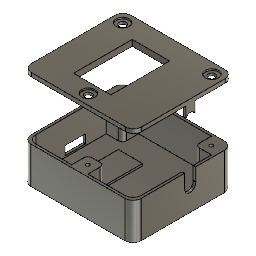
ScopeControl-fusion360 (Autodesk Fusion 360 design; units mm, degrees)
Autodesk Fusion 360 part; units mm, degrees
sketch "Sketch1" plane through (0, 0, 0) normal (0, 0, 1) x (1, 0, 0)
  line L0 (0, 0) -> (54.6, 0)
  line L1 (54.6, 0) -> (54.6, -49.3)
  line L2 (54.6, -49.3) -> (0, -49.3)
  line L3 (0, -49.3) -> (0, 0)
  dimension "d1" = 54.6
  dimension "d2" = 49.3
  constraint horizontal L0
  constraint vertical L1
  constraint horizontal L2
  constraint vertical L3
  constraint coincident L0.start L3.end
  measures "d1" distance of L0.start L0.end
  measures "d2" distance of L0.start L2.end
extrude "Extrude1" add sketch "Sketch1" along normal blind 1.25 makes body 1
sketch "Sketch2" plane through (0, 0, 1.25) normal (0, 0, 1) x (-1, 0, 0)
  line L0 (0, 49.3) -> (-54.6, 49.3)
  line L1 (-54.6, 49.3) -> (-54.6, 0)
  line L2 (-54.6, 0) -> (0, 0)
  line L3 (0, 0) -> (0, 49.3)
  line L4 (-1.25, 48.05) -> (-53.35, 48.05)
  line L5 (-53.35, 48.05) -> (-53.35, 1.25)
  line L6 (-53.35, 1.25) -> (-1.25, 1.25)
  line L7 (-1.25, 1.25) -> (-1.25, 48.05)
  dimension "d5" = -1.25
extrude "Extrude2" add sketch "Sketch2" along normal blind 17.5 bodies 1
sketch "Sketch3" plane through (0, 0, 1.25) normal (0, 0, 1) x (-1, 0, 0)
  line L0 (-1.25, 48.05) -> (-53.35, 48.05)
  line L1 (-53.35, 48.05) -> (-53.35, 1.25)
  line L2 (-53.35, 1.25) -> (-1.25, 1.25)
  line L3 (-1.25, 1.25) -> (-1.25, 48.05)
  line L4 (-1.25, 1.25) -> (-9.25, 1.25)
  line L5 (-9.25, 1.25) -> (-9.25, 9.25)
  line L6 (-9.25, 9.25) -> (-1.25, 9.25)
  line L7 (-1.25, 9.25) -> (-1.25, 1.25)
  dimension "d8" = 8
  dimension "d9" = 8
  constraint horizontal L4
  constraint vertical L5
  constraint horizontal L6
  constraint vertical L7
  constraint coincident L2.end L3.start
  measures "d8" distance of L2.end L4.end
  measures "d9" distance of L2.end L6.end
extrude "Extrude3" add sketch "Sketch3" along normal blind 17.5 contours L2 L3 L4 L5 L6 L7 bodies 1
sketch "Sketch4" plane through (0, 0, 1.25) normal (0, 0, 1) x (-1, 0, 0)
  line L0 (-9.25, 1.25) -> (-9.25, 9.25)
  line L1 (-9.25, 9.25) -> (-1.25, 9.25)
  line L2 (-1.25, 9.25) -> (-1.25, 48.05)
  line L3 (-1.25, 48.05) -> (-53.35, 48.05)
  line L4 (-53.35, 48.05) -> (-53.35, 1.25)
  line L5 (-53.35, 1.25) -> (-9.25, 1.25)
  line L6 (-53.35, 1.25) -> (-45.35, 1.25)
  line L7 (-45.35, 1.25) -> (-45.35, 9.25)
  line L8 (-45.35, 9.25) -> (-53.35, 9.25)
  line L9 (-53.35, 9.25) -> (-53.35, 1.25)
  dimension "d12" = 8
  dimension "d13" = 8
  constraint horizontal L6
  constraint vertical L7
  constraint horizontal L8
  constraint vertical L9
  constraint coincident L4.end L5.start
  measures "d12" distance of L4.end L6.end
  measures "d13" distance of L4.end L8.end
extrude "Extrude4" add sketch "Sketch4" along normal blind 17.5 contours L4 L5 L6 L7 L8 L9 bodies 1
sketch "Sketch5" plane through (0, 0, 1.25) normal (0, 0, 1) x (-1, 0, 0)
  line L0 (-45.35, 9.25) -> (-45.35, 1.25)
  line L1 (-45.35, 1.25) -> (-9.25, 1.25)
  line L2 (-9.25, 1.25) -> (-9.25, 9.25)
  line L3 (-9.25, 9.25) -> (-1.25, 9.25)
  line L4 (-1.25, 9.25) -> (-1.25, 48.05)
  line L5 (-1.25, 48.05) -> (-53.35, 48.05)
  line L6 (-53.35, 48.05) -> (-53.35, 9.25)
  line L7 (-53.35, 9.25) -> (-45.35, 9.25)
  line L8 (-22.9932, 48.05) -> (-30.9932, 48.05)
  line L9 (-30.9932, 48.05) -> (-30.9932, 40.05)
  line L10 (-30.9932, 40.05) -> (-22.9932, 40.05)
  line L11 (-22.9932, 40.05) -> (-22.9932, 48.05)
  dimension "d16" = 8
  dimension "d17" = 8
  constraint horizontal L8
  constraint vertical L9
  constraint horizontal L10
  constraint vertical L11
  constraint coincident L5 L8.start
  measures "d16" distance of L8.start L8.end
  measures "d17" distance of L8.start L10.end
extrude "Extrude5" add sketch "Sketch5" along normal blind 17.5 contours L5 L8 L9 L10 L11 bodies 1
sketch "Sketch6" plane through (0, 0, 0) normal (-1, 0, 0) x (0, -1, 0)
  line L0 (0, 0) -> (49.3, 0)
  line L1 (49.3, 0) -> (49.3, 18.75)
  line L2 (49.3, 18.75) -> (0, 18.75)
  line L3 (0, 18.75) -> (0, 0)
  line L4 (19.5046, 2.0157) -> (29.5046, 2.0157)
  line L5 (29.5046, 2.0157) -> (29.5046, 6.3157)
  line L6 (29.5046, 6.3157) -> (19.5046, 6.3157)
  line L7 (19.5046, 6.3157) -> (19.5046, 2.0157)
  dimension "d20" = 10
  dimension "d21" = 4.3
  constraint horizontal L4
  constraint vertical L5
  constraint horizontal L6
  constraint vertical L7
  measures "d20" distance of L4.start L4.end
  measures "d21" distance of L4.start L6.end
extrude "Extrude6" cut sketch "Sketch6" against normal blind 2 contours L4 L5 L6 L7 bodies 1
sketch "Sketch7" plane through (54.6, 0, 0) normal (1, 0, 0) x (0, 1, 0)
  line L0 (-49.3, 0) -> (0, 0)
  line L1 (0, 0) -> (0, 18.75)
  line L2 (0, 18.75) -> (-49.3, 18.75)
  line L3 (-49.3, 18.75) -> (-49.3, 0)
  circle A0 centre (-21.0556, 11.4278) radius 2.75
  dimension "d24" = 5.5
  measures "d24" diameter of A0
extrude "Extrude7" cut sketch "Sketch7" against normal blind 2 contours A0 bodies 1
sketch "Sketch8" plane through (0, 0, 1.25) normal (0, 0, 1) x (-1, 0, 0)
  line L0 (-30.9932, 40.05) -> (-30.9932, 48.05)
  line L1 (-30.9932, 48.05) -> (-53.35, 48.05)
  line L2 (-53.35, 48.05) -> (-53.35, 9.25)
  line L3 (-53.35, 9.25) -> (-45.35, 9.25)
  line L4 (-45.35, 9.25) -> (-45.35, 1.25)
  line L5 (-45.35, 1.25) -> (-9.25, 1.25)
  line L6 (-9.25, 1.25) -> (-9.25, 9.25)
  line L7 (-9.25, 9.25) -> (-1.25, 9.25)
  line L8 (-1.25, 9.25) -> (-1.25, 48.05)
  line L9 (-1.25, 48.05) -> (-22.9932, 48.05)
  line L10 (-22.9932, 48.05) -> (-22.9932, 40.05)
  line L11 (-22.9932, 40.05) -> (-30.9932, 40.05)
  line L12 (-12, 14) -> (-24, 14)
  line L13 (-24, 14) -> (-24, 36)
  line L14 (-24, 36) -> (-12, 36)
  line L15 (-12, 36) -> (-12, 14)
  dimension "d27" = 12
  dimension "d28" = 22
  constraint horizontal L12
  constraint vertical L13
  constraint horizontal L14
  constraint vertical L15
  measures "d27" distance of L12.start L12.end
  measures "d28" distance of L12.start L14.end
extrude "Extrude8" add sketch "Sketch8" along normal blind 1 contours L12 L13 L14 L15 bodies 1
sketch "Sketch9" plane through (0, 0, 18.75) normal (0, 0, 1) x (-1, 0, 0)
  line L0 (-1.25, 48.05) -> (-1.25, 9.25)
  line L1 (-1.25, 9.25) -> (-9.25, 9.25)
  line L2 (-9.25, 9.25) -> (-9.25, 1.25)
  line L3 (-9.25, 1.25) -> (-45.35, 1.25)
  line L4 (-45.35, 1.25) -> (-45.35, 9.25)
  line L5 (-45.35, 9.25) -> (-53.35, 9.25)
  line L6 (-53.35, 9.25) -> (-53.35, 48.05)
  line L7 (-53.35, 48.05) -> (-30.9932, 48.05)
  line L8 (-30.9932, 48.05) -> (-30.9932, 40.05)
  line L9 (-30.9932, 40.05) -> (-22.9932, 40.05)
  line L10 (-22.9932, 40.05) -> (-22.9932, 48.05)
  line L11 (-22.9932, 48.05) -> (-1.25, 48.05)
  line L12 (0, 0) -> (0, 49.3)
  line L13 (0, 49.3) -> (-54.6, 49.3)
  line L14 (-54.6, 49.3) -> (-54.6, 0)
  line L15 (-54.6, 0) -> (0, 0)
  line L16 (0, 0) -> (-54.6, 0)
  line L17 (-54.6, 0) -> (-54.6, 49.3)
  line L18 (-54.6, 49.3) -> (0, 49.3)
  line L19 (0, 49.3) -> (0, 0)
  constraint horizontal L16
  constraint vertical L17
  constraint horizontal L18
  constraint vertical L19
  constraint coincident L13.end L14.start
  constraint coincident L12.start L15.end
extrude "Extrude1'" add sketch "Sketch9" along normal blind 2 separate body contours L0 L1 L2 L3 L4 L5 L6 L7 L8 L9 L10 L11 | L12 L13 L14 L15 L16 L17 L18 L19 makes body 2 in component "Lid"
hole "Hole1" at (26.9994, -44.0897, 20.75) direction (0, 0, -1) diameter 1.8 depth 10 tip angle 118 bodies 1
hole "Hole1'" at (26.9994, -44.0897, 20.75) direction (0, 0, -1) diameter 1.8 depth 10 tip angle 118 bodies 2 in component "Lid"
sketch "Sketch10" plane through (0, 0, 20.75) normal (0, 0, 1) x (-1, 0, 0)
  circle A0 centre (-26.9994, 44.0897) radius 0.9
  line L0 (0, 49.3) -> (-54.6, 49.3)
  line L1 (-54.6, 49.3) -> (-54.6, 0)
  line L2 (-54.6, 0) -> (0, 0)
  line L3 (0, 0) -> (0, 49.3)
  circle A1 centre (-26.9994, 44.0897) radius 1.75
  dimension "d39" = 3.5
  constraint concentric A0 A1
  measures "d39" diameter of A1
extrude "Extrude2'" cut sketch "Sketch10" against normal blind 2 contours A1 bodies 2 in component "Lid"
sketch "Sketch11" plane through (0, 0, 20.75) normal (0, 0, 1) x (-1, 0, 0)
  circle A0 centre (-26.9994, 44.0897) radius 1.75
  line L0 (0, 49.3) -> (-54.6, 49.3)
  line L1 (-54.6, 49.3) -> (-54.6, 0)
  line L2 (-54.6, 0) -> (0, 0)
  line L3 (0, 0) -> (0, 49.3)
  circle A1 centre (-26.9994, 44.0897) radius 3.25
  dimension "d42" = 6.5
  constraint concentric A0 A1
  measures "d42" diameter of A1
extrude "Extrude3'" cut sketch "Sketch11" against normal blind 0.75 contours A1 bodies 2 in component "Lid"
hole "Hole2" at (5.1718, -5.2287, 18.75) direction (0, 0, -1) diameter 1.8 depth 10 tip angle 118 bodies 1
hole "Hole3" at (49.3508, -5.29, 18.75) direction (0, 0, -1) diameter 1.8 depth 10 tip angle 118 bodies 1
hole "Hole2'" at (5.1718, -5.29, 20.75) direction (0, 0, -1) diameter 3.5 depth 2 tip angle 180 counterbore diameter 6.5 counterbore depth 0.75 bodies 2 in component "Lid"
hole "Hole3'" at (49.3508, -5.29, 20.75) direction (0, 0, -1) diameter 3.5 depth 2 tip angle 180 counterbore diameter 6.5 counterbore depth 0.75 bodies 2 in component "Lid"
fillet "Fillet1" radius 4 1 edges at (54.6, -49.3, 9.375) on bodies 1
fillet "Fillet1'" radius 4 1 edges at (54.6, -49.3, 19.75) on bodies 2 in component "Lid"
fillet "Fillet2" radius 4 1 edges at (54.6, 0, 9.375) on bodies 1
fillet "Fillet2'" radius 4 1 edges at (54.6, 0, 19.75) on bodies 2 in component "Lid"
fillet "Fillet3" radius 4 1 edges at (0, -49.3, 9.375) on bodies 1
fillet "Fillet3'" radius 4 1 edges at (0, -49.3, 19.75) on bodies 2 in component "Lid"
fillet "Fillet4" radius 4 1 edges at (0, 0, 9.375) on bodies 1
fillet "Fillet4'" radius 4 1 edges at (0, 0, 19.75) on bodies 2 in component "Lid"
fillet "Fillet5" radius 2 1 edges at (9.25, -9.25, 10) on bodies 1
fillet "Fillet6" radius 2 1 edges at (45.35, -9.25, 10) on bodies 1
fillet "Fillet7" radius 2 1 edges at (30.9932, -40.05, 10) on bodies 1
fillet "Fillet8" radius 2 1 edges at (22.9932, -40.05, 10) on bodies 1
fillet "Fillet9" radius 4 1 edges at (1.25, -48.05, 10) on bodies 1
fillet "Fillet10" radius 4 1 edges at (53.35, -48.05, 10) on bodies 1
ref_plane "WorkPlane1" through (27.3, -24.65, 19.75) normal (0, 1, 0) x (-1, 0, 0)
ref_plane "WorkPlane2" through (24, -24.65, 19.75) normal (-1, 0, 0) x (0, -1, 0)
sketch "Sketch12" plane through (0, 0, 20.75) normal (0, 0, 1) x (-1, 0, 0)
  arc A0 (-4, 0) -> (0, 4) centre (-4, 4) ccw
  line L0 (0, 4) -> (0, 45.3)
  arc A1 (0, 45.3) -> (-4, 49.3) centre (-4, 45.3) ccw
  line L1 (-4, 49.3) -> (-50.6, 49.3)
  arc A2 (-50.6, 49.3) -> (-54.6, 45.3) centre (-50.6, 45.3) ccw
  line L2 (-54.6, 45.3) -> (-54.6, 4)
  arc A3 (-54.6, 4) -> (-50.6, 0) centre (-50.6, 4) ccw
  line L3 (-50.6, 0) -> (-4, 0)
  circle A4 centre (-49.3508, 5.29) radius 3.25
  circle A5 centre (-5.1718, 5.29) radius 3.25
  circle A6 centre (-26.9994, 44.0897) radius 3.25
  line L4 (-31.7409, 37.6384) -> (-16.2409, 37.6384)
  line L5 (-16.2409, 37.6384) -> (-16.2409, 11.6384)
  line L6 (-16.2409, 11.6384) -> (-31.7409, 11.6384)
  line L7 (-31.7409, 11.6384) -> (-31.7409, 37.6384)
  line L8 (-31.7409, 37.6384) -> (-16.2409, 11.6384) construction
  line L9 (-16.2409, 37.6384) -> (-31.7409, 11.6384) construction
  point P0 (-23.9909, 24.6384)
  dimension "d90" = 15.5
  dimension "d91" = 26
  constraint horizontal L4
  constraint perpendicular L4 L5
  constraint parallel L4 L6
  constraint parallel L5 L7
  constraint coincident L8 P0
  constraint coincident L9 P0
  measures "d90" distance of L5.end L6.end
  measures "d91" distance of L4.end L5.end
extrude "Extrude4'" cut sketch "Sketch12" against normal blind 2 contours L4 L5 L6 L7 bodies 2 in component "Lid"
sketch "Sketch13" plane through (0, 0, 18.75) normal (0, 0, -1) x (1, 0, 0)
  line L0 (16.2409, 11.6384) -> (16.2409, 37.6384)
  line L1 (16.2409, 37.6384) -> (31.7409, 37.6384)
  line L2 (31.7409, 37.6384) -> (31.7409, 11.6384)
  line L3 (31.7409, 11.6384) -> (16.2409, 11.6384)
  circle A0 centre (49.3508, 5.29) radius 1.75
  circle A1 centre (5.1718, 5.29) radius 1.75
  circle A2 centre (26.9994, 44.0897) radius 1.75
  arc A3 (0, 4) -> (4, 0) centre (4, 4) ccw
  line L4 (4, 0) -> (50.6, 0)
  arc A4 (50.6, 0) -> (54.6, 4) centre (50.6, 4) ccw
  line L5 (54.6, 4) -> (54.6, 45.3)
  arc A5 (54.6, 45.3) -> (50.6, 49.3) centre (50.6, 45.3) ccw
  line L6 (50.6, 49.3) -> (4, 49.3)
  arc A6 (4, 49.3) -> (0, 45.3) centre (4, 45.3) ccw
  line L7 (0, 45.3) -> (0, 4)
  line L8 (8, 40) -> (45.675, 40)
  line L9 (45.675, 40) -> (45.675, 9.5543)
  line L10 (45.675, 9.5543) -> (8, 9.5543)
  line L11 (8, 9.5543) -> (8, 40)
  constraint horizontal L8
  constraint vertical L9
  constraint horizontal L10
  constraint vertical L11
extrude "Extrude5'" cut sketch "Sketch13" against normal blind 0.5 contours L8 L9 L10 L11 bodies 2 in component "Lid"
chamfer "Chamfer1" distance 1.5 angle 45 4 edges at (23.9909, -11.6384, 20.75) (16.2409, -24.6384, 20.75) (23.9909, -37.6384, 20.75) (31.7409, -24.6384, 20.75) on bodies 2 in component "Lid"
extrude "Extrude9" cut 1 faces at (48.3618, -1.8887, 18.75) along direction (0, 0, -1) blind 0.5 on bodies 1 bodies 1
ref_plane "WorkPlane3" through (54.2337, -23.8056, 11.4278) normal (0, 1, 0) x (0, 0, 1)
ref_plane "WorkPlane4" through (54.0778, -18.3056, 11.4278) normal (0, -1, 0) x (0, 0, -1)
sketch "Sketch14" plane through (0, 0, 18.25) normal (0, 0, 1) x (-1, 0, 0)
  circle A0 centre (-49.3508, 5.29) radius 0.9
  circle A1 centre (-5.1718, 5.2287) radius 0.9
  circle A2 centre (-26.9994, 44.0897) radius 0.9
  arc A3 (-24.9932, 40.05) -> (-22.9932, 42.05) centre (-24.9932, 42.05) ccw
  line L0 (-22.9932, 42.05) -> (-22.9932, 48.05)
  line L1 (-22.9932, 48.05) -> (-5.25, 48.05)
  arc A4 (-1.25, 44.05) -> (-5.25, 48.05) centre (-5.25, 44.05) ccw
  line L2 (-1.25, 44.05) -> (-1.25, 9.25)
  line L3 (-1.25, 9.25) -> (-7.25, 9.25)
  arc A5 (-7.25, 9.25) -> (-9.25, 7.25) centre (-7.25, 7.25) ccw
  line L4 (-9.25, 7.25) -> (-9.25, 1.25)
  line L5 (-9.25, 1.25) -> (-45.35, 1.25)
  line L6 (-45.35, 1.25) -> (-45.35, 7.25)
  arc A6 (-45.35, 7.25) -> (-47.35, 9.25) centre (-47.35, 7.25) ccw
  line L7 (-47.35, 9.25) -> (-53.35, 9.25)
  line L8 (-53.35, 9.25) -> (-53.35, 44.05)
  arc A7 (-49.35, 48.05) -> (-53.35, 44.05) centre (-49.35, 44.05) ccw
  line L9 (-49.35, 48.05) -> (-30.9932, 48.05)
  line L10 (-30.9932, 48.05) -> (-30.9932, 42.05)
  arc A8 (-30.9932, 42.05) -> (-28.9932, 40.05) centre (-28.9932, 42.05) ccw
  line L11 (-28.9932, 40.05) -> (-24.9932, 40.05)
  arc A9 (-4, 0) -> (0, 4) centre (-4, 4) ccw
  line L12 (0, 4) -> (0, 45.3)
  arc A10 (0, 45.3) -> (-4, 49.3) centre (-4, 45.3) ccw
  line L13 (-4, 49.3) -> (-50.6, 49.3)
  arc A11 (-50.6, 49.3) -> (-54.6, 45.3) centre (-50.6, 45.3) ccw
  line L14 (-54.6, 45.3) -> (-54.6, 4)
  arc A12 (-54.6, 4) -> (-50.6, 0) centre (-50.6, 4) ccw
  line L15 (-50.6, 0) -> (-4, 0)
  line L16 (-53.35, 18.332) -> (-54.6, 18.332)
  line L17 (-54.6, 18.332) -> (-54.6, 23.8049)
  line L18 (-54.6, 23.8049) -> (-53.35, 23.8049)
  line L19 (-53.35, 23.8049) -> (-53.35, 18.332)
  constraint horizontal L16
  constraint vertical L17
  constraint horizontal L18
  constraint vertical L19
  constraint coincident L14 L17.end
  constraint coincident L8 L16.start
extrude "Extrude10" cut sketch "Sketch14" against normal blind 6.7 contours L8 L14 L16 L17 L18 L19 bodies 1
sketch "Sketch15" plane through (0, 0, 20.75) normal (0, 0, 1) x (-1, 0, 0)
  circle A0 centre (-26.9994, 44.0897) radius 3.25
  circle A1 centre (-5.1718, 5.29) radius 3.25
  circle A2 centre (-49.3508, 5.29) radius 3.25
  arc A3 (-4, 0) -> (0, 4) centre (-4, 4) ccw
  line L0 (0, 4) -> (0, 45.3)
  arc A4 (0, 45.3) -> (-4, 49.3) centre (-4, 45.3) ccw
  line L1 (-4, 49.3) -> (-50.6, 49.3)
  arc A5 (-50.6, 49.3) -> (-54.6, 45.3) centre (-50.6, 45.3) ccw
  line L2 (-54.6, 45.3) -> (-54.6, 4)
  arc A6 (-54.6, 4) -> (-50.6, 0) centre (-50.6, 4) ccw
  line L3 (-50.6, 0) -> (-4, 0)
  line L4 (-33.2409, 39.1384) -> (-14.7409, 39.1384)
  line L5 (-14.7409, 39.1384) -> (-14.7409, 10.1384)
  line L6 (-14.7409, 10.1384) -> (-33.2409, 10.1384)
  line L7 (-33.2409, 10.1384) -> (-33.2409, 39.1384)
  line L8 (-54.6, 18.7295) -> (-53.35, 18.7295)
  line L9 (-53.35, 18.7295) -> (-53.35, 23.4295)
  line L10 (-53.35, 23.4295) -> (-54.6, 23.4295)
  line L11 (-54.6, 23.4295) -> (-54.6, 18.7295)
  dimension "d103" = 1.25
  dimension "d104" = 4.7
  constraint horizontal L8
  constraint vertical L9
  constraint horizontal L10
  constraint vertical L11
  constraint coincident L2 L8.start
  measures "d103" distance of L8.start L8.end
  measures "d104" distance of L8.start L10.end
extrude "Extrude6'" add sketch "Sketch15" against normal blind 8.8 contours L2 L8 L9 L10 L11 bodies 2 in component "Lid"
sketch "Sketch16" plane through (54.6, 0, 0) normal (1, 0, 0) x (0, 1, 0)
  line L0 (-4, 20.75) -> (-45.3, 20.75)
  line L1 (-45.3, 20.75) -> (-45.3, 18.75)
  line L2 (-45.3, 18.75) -> (-23.4295, 18.75)
  line L3 (-23.4295, 18.75) -> (-23.4295, 11.95)
  line L4 (-23.4295, 11.95) -> (-18.7295, 11.95)
  line L5 (-18.7295, 11.95) -> (-18.7295, 18.75)
  line L6 (-18.7295, 18.75) -> (-4, 18.75)
  line L7 (-4, 18.75) -> (-4, 20.75)
  circle A0 centre (-21.1349, 12.3888) radius 2.5191
extrude "Extrude7'" cut sketch "Sketch16" against normal blind 1.5 contours L3 L4 L5 A0 picked at (-20.6526, 12.8081) bodies 2 in component "Lid"
move_body "Move1" bodies 2 to x (1, 0, 0) y (0, -1, 0) z (0, 0, -1) at (0, 40.8197, 28.5) in component "Lid"
move_body "Move2" bodies 2 to x (1, 0, 0) y (0, 1, 0) z (0, 0, 1) at (0, 0, -8) in component "Lid"
move_body "Move3" bodies 2 to x (1, 0, 0) y (0, 1, 0) z (0, 0, 1) at (0, -23, 0) in component "Lid"
move_body "Move4" bodies 2 to x (1, 0, 0) y (0, 1, 0) z (0, 0, 1) at (0, -8, 0) in component "Lid"
move_body "Move5" bodies 2 to x (1, 0, 0) y (0, -1, 0) z (0, 0, -1) at (0, 107.0872, 29.5) in component "Lid"
move_body "Move6" bodies 2 to x (1, 0, 0) y (0, 1, 0) z (0, 0, 1) at (0, -97, 19) in component "Lid"
component "Lid" placed x (1, 0, 0) y (0, 1, 0) z (0, 0, 1) at (0, 0, 0)
